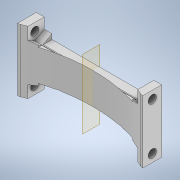
# Autodesk Inventor part: InnerSpacer
Saved by Autodesk Inventor 2020 (Build 240168000, 168)
## iProperties
Created: 2020-02-08
Part Number: InnerSpacer
Material: Generic
Document SubType Name: Modeling
Designer: srini
Density: 1 g/cm^3
Appearance: Default
Author: srini
Autodesk Inventor part; units mm, degrees
ref_plane "YZ Plane" through (0, 0, 0) normal (1, 0, 0) x (0, 1, 0)
ref_plane "XZ Plane" through (0, 0, 0) normal (0, 1, 0) x (-1, 0, 0)
ref_plane "XY Plane" through (0, 0, 0) normal (0, 0, 1) x (1, 0, 0)
sketch "Sketch1" plane through (0, 0, 0) normal (0, 0, 1) x (1, 0, 0)
  line L0 (-50.8, 12.7) -> (50.8, 12.7)
  line L1 (50.8, 12.7) -> (50.8, -12.7)
  line L2 (50.8, -12.7) -> (-50.8, -12.7)
  line L3 (-50.8, -12.7) -> (-50.8, 12.7)
  line L4 (-50.8, 25.4) -> (-38.1, 25.4)
  line L5 (-38.1, 25.4) -> (-38.1, 12.7)
  line L6 (-38.1, 12.7) -> (-50.8, 12.7)
  line L7 (-50.8, 12.7) -> (-50.8, 25.4)
  line L8 (-50.8, -12.7) -> (-38.1, -12.7)
  line L9 (-38.1, -12.7) -> (-38.1, -25.4)
  line L10 (-38.1, -25.4) -> (-50.8, -25.4)
  line L11 (-50.8, -25.4) -> (-50.8, -12.7)
  line L12 (38.1, 25.4) -> (50.8, 25.4)
  line L13 (50.8, 25.4) -> (50.8, 12.7)
  line L14 (50.8, 12.7) -> (38.1, 12.7)
  line L15 (38.1, 12.7) -> (38.1, 25.4)
  line L16 (38.1, -12.7) -> (50.8, -12.7)
  line L17 (50.8, -12.7) -> (50.8, -25.4)
  line L18 (50.8, -25.4) -> (38.1, -25.4)
  line L19 (38.1, -25.4) -> (38.1, -12.7)
  point P0 (0, 0)
  point P1 (-38.1, -12.7)
  point P2 (38.1, -12.7)
  dimension "d0" = 101.6
  dimension "d1" = 50.8
  dimension "d2" = 25.4
  dimension "d3" = 12.7
  dimension "d4" = 12.7
  dimension "d5" = 12.7
  constraints: 40 end point, 10 parallel, 7 collinear, 6 equal length, 5 horizontal, 5 perpendicular, 1 point on line
  measures "d0" distance of L0.start L0.end
  measures "d1" distance from line of point (0, 0) L3
  measures "d2" distance between parallel lines of L2 L0
  measures "d3" distance from line of point (0, 0) L0
  measures "d4" distance of L4.start L4.end
  measures "d5" distance of L6.end L4.start
extrude "Extrusion1" add sketch "Sketch1" along normal blind 15.24
sketch "Sketch2" plane through (50.8, -25.4, 0) normal (1, 0, 0) x (0, 0, -1)
  circle A0 centre (-7.62, 44.45) radius 3.3734
  line L0 (0, 0) -> (0, 50.8) projected
  line L1 (0, 50.8) -> (-15.24, 50.8) projected
  circle A1 centre (-7.62, 6.35) radius 3.3734
  point P0 (0, 25.4)
  dimension "d8" = 7.62
  dimension "d9" = 6.35
  dimension "d10" = 6.7469
  dimension "d13" = 38.1
  constraints: 2 centre point, 1 vertical, 2 other
  measures "d8" distance from line of A0.centre L0
  measures "d9" distance from line of A0.centre L1
  measures "d10" diameter of A0
  measures "d13" distance of A0.centre A1.centre
extrude "Extrusion2" cut sketch "Sketch2" against normal through all
sketch "Sketch3" plane through (-38.1, 12.7, 0) normal (1, 0, 0) x (0, 0, -1)
  circle A0 centre (-7.62, 6.35) radius 3.3734 projected
  circle A1 centre (-7.62, -31.75) radius 3.3734 projected
  line L0 (-7.62, 12.9967) -> (-1.8638, 9.6734)
  line L1 (-1.8638, 9.6734) -> (-1.8638, 3.0266)
  line L2 (-1.8638, 3.0266) -> (-7.62, -0.2967)
  line L3 (-7.62, -0.2967) -> (-13.3762, 3.0266)
  line L4 (-13.3762, 3.0266) -> (-13.3763, 9.6734)
  line L5 (-13.3763, 9.6734) -> (-7.62, 12.9967)
  line L6 (-7.62, -25.1033) -> (-1.8638, -28.4266)
  line L7 (-1.8638, -28.4266) -> (-1.8638, -35.0734)
  line L8 (-1.8638, -35.0734) -> (-7.62, -38.3967)
  line L9 (-7.62, -38.3967) -> (-13.3762, -35.0734)
  line L10 (-13.3762, -35.0734) -> (-13.3762, -28.4266)
  line L11 (-13.3762, -28.4266) -> (-7.62, -25.1033)
  point P0 (0, -12.7)
  point P1 (-7.62, 6.35)
  point P2 (-7.62, -31.75)
  dimension "d20" = 11.5125
  constraints: 24 end point, 2 coincident, 1 equal length, 1 vertical, 1 vertical alignment, 26 other
  measures "d20" distance between parallel lines of L4 L1
extrude "Extrusion3" cut sketch "Sketch3" against normal blind 6.35 contours A0 | A1 | L0 L1 L2 L3 L4 L5 | L6 L7 L8 L9 L10 L11
ref_plane "Work Plane1" through (0, -25.4, 0) normal (1, 0, 0) x (0, 0, -1)
mirror "Mirror1" about plane through (0, -25.4, 0) normal (1, 0, 0) of "Extrusion3"
sketch "Sketch4" plane through (-38.1, -12.7, 0) normal (0, -1, 0) x (1, 0, 0)
  circle A0 centre (38.1, 132.08) radius 127
  line L0 (0, 0) -> (76.2, 0) projected
  point P0 (38.1, 0)
  point P1 (38.1, 0)
  dimension "d23" = 132.08
  dimension "d24" = 254
  constraints: 1 centre point, 1 midpoint, 1 vertical alignment
  measures "d23" distance of point (38.1, 0) A0.centre
  measures "d24" diameter of A0
extrude "Extrusion4" cut sketch "Sketch4" against normal through all both and the other way through all
fillet "Fillet1" radius 6.35 2 edges at (49.7736, 0, 15.24) (-49.7736, 0, 15.24)
sketch "Sketch5" plane through (0, 0, 0) normal (0, 0, -1) x (-1, 0, 0)
  line L0 (-25.4, 9.525) -> (25.4, 9.525) construction
  line L1 (25.4, 9.525) -> (25.4, -9.525) construction
  line L2 (25.4, -9.525) -> (-25.4, -9.525) construction
  line L3 (-25.4, -9.525) -> (-25.4, 9.525) construction
  spline S0 degree 2 poles (-27.0681, 4.7718) (-25.0031, 4.7718) (-22.4544, 2.2603) (-22.4544, -0.0279) knots 0 0 0 1 2 2 2
  line L4 (-22.4544, -0.0279) -> (-22.4544, -9.9064)
  line L5 (-22.4544, -9.9064) -> (-24.4822, -9.9064)
  line L6 (-24.4822, -9.9064) -> (-24.4822, -0.1953)
  spline S1 degree 2 poles (-24.4822, -0.1953) (-24.4822, 1.4976) (-26.0635, 3.1347) (-27.496, 3.1347) knots 0 0 0 1 2 2 2
  spline S2 degree 2 poles (-27.496, 3.1347) (-30.0261, 3.1347) (-31.6074, 0.5674) knots 0 0 0 1 1 1
  line L7 (-31.6074, 0.5674) -> (-31.6074, -9.9064)
  line L8 (-31.6074, -9.9064) -> (-33.6166, -9.9064)
  line L9 (-33.6166, -9.9064) -> (-33.6166, 10.2412)
  line L10 (-33.6166, 10.2412) -> (-31.6074, 10.2412)
  line L11 (-31.6074, 10.2412) -> (-31.6074, 2.6138)
  spline S3 degree 2 poles (-31.6074, 2.6138) (-29.9703, 4.7718) (-27.0681, 4.7718) knots 0 0 0 1 1 1
  line L12 (-7.7019, -4.0277) -> (-15.1247, -4.0277)
  line L13 (-15.1247, -4.0277) -> (-16.985, -9.9064)
  line L14 (-16.985, -9.9064) -> (-19.0686, -9.9064)
  line L15 (-19.0686, -9.9064) -> (-12.8364, 9.1436)
  line L16 (-12.8364, 9.1436) -> (-10.0273, 9.1436)
  line L17 (-10.0273, 9.1436) -> (-3.6091, -9.9064)
  line L18 (-3.6091, -9.9064) -> (-5.7299, -9.9064)
  line L19 (-5.7299, -9.9064) -> (-7.7019, -4.0277)
  line L20 (-14.6038, -2.3347) -> (-8.2414, -2.3347)
  line L21 (-8.2414, -2.3347) -> (-11.4598, 7.6553)
  line L22 (-11.4598, 7.6553) -> (-14.6038, -2.3347)
  line L23 (10.9761, 7.5995) -> (0.9488, -8.2135)
  line L24 (0.9488, -8.2135) -> (11.1993, -8.2135)
  line L25 (11.1993, -8.2135) -> (11.1993, -9.9064)
  line L26 (11.1993, -9.9064) -> (-1.3209, -9.9064)
  line L27 (-1.3209, -9.9064) -> (-1.3209, -8.3065)
  line L28 (-1.3209, -8.3065) -> (8.725, 7.4879)
  line L29 (8.725, 7.4879) -> (-0.893, 7.4879)
  line L30 (-0.893, 7.4879) -> (-0.893, 9.1436)
  line L31 (-0.893, 9.1436) -> (10.9761, 9.1436)
  line L32 (10.9761, 9.1436) -> (10.9761, 7.5995)
  line L33 (17.878, 7.4879) -> (17.878, 0.7348)
  line L34 (17.878, 0.7348) -> (25.5426, 0.7348)
  line L35 (25.5426, 0.7348) -> (25.5426, -0.9581)
  line L36 (25.5426, -0.9581) -> (17.878, -0.9581)
  line L37 (17.878, -0.9581) -> (17.878, -8.2507)
  line L38 (17.878, -8.2507) -> (26.1379, -8.2507)
  line L39 (26.1379, -8.2507) -> (26.1379, -9.9064)
  line L40 (26.1379, -9.9064) -> (15.8316, -9.9064)
  line L41 (15.8316, -9.9064) -> (15.8316, 9.1436)
  line L42 (15.8316, 9.1436) -> (26.1379, 9.1436)
  line L43 (26.1379, 9.1436) -> (26.1379, 7.4879)
  line L44 (26.1379, 7.4879) -> (17.878, 7.4879)
  spline S4 degree 2 poles (32.8538, -7.2647) (32.8538, -7.9716) (33.4119, -8.5669) (34.0072, -8.5669) knots 0 0 0 1 2 2 2
  spline S5 degree 2 poles (34.0072, -8.5669) (34.4351, -8.5669) (34.8444, -8.4553) knots 0 0 0 1 1 1
  line L45 (34.8444, -8.4553) -> (35.1234, -9.9064)
  spline S6 degree 2 poles (35.1234, -9.9064) (34.3235, -10.2412) (33.4863, -10.2412) knots 0 0 0 1 1 1
  spline S7 degree 2 poles (33.4863, -10.2412) (32.2585, -10.2412) (30.8446, -8.846) (30.8446, -7.5623) knots 0 0 0 1 2 2 2
  line L46 (30.8446, -7.5623) -> (30.8446, 10.2412)
  line L47 (30.8446, 10.2412) -> (32.8538, 10.2412)
  line L48 (32.8538, 10.2412) -> (32.8538, -7.2647)
  point P0 (0, 0)
  dimension "d2" = 25.4
  dimension "d30" = 50.8
  dimension "d31" = 25.4
  dimension "d32" = 19.05
  dimension "d33" = 9.525
  constraints: 2 other
  measures "d30" distance of L0.start L0.end
  measures "d31" distance from line of point (0, 0) L3
  measures "d32" distance of L0.end L1.end
  measures "d33" distance from line of point (0, 0) L0
emboss "Emboss1" sketch "Sketch5" operation cut depth 0.9 direction (0, 0, 1)
sketch "Sketch6" plane through (44.45, 15.7266, 13.3762) normal (-1, 0, 0) x (0, 1, 0)
  point P0 (-15.7266, 13.3762)
sketch "Sketch7" plane through (-44.45, 12.7, 0) normal (1, 0, 0) x (0, 0, -1)
  line L0 (-7.62, -0.2967) -> (-18.6172, 6.0525)
  line L1 (-18.6172, 6.0525) -> (-19.0863, 27.5679)
  line L2 (-19.0863, 27.5679) -> (7.0141, 38.5627)
  line L3 (7.0141, 38.5627) -> (10.8216, 10.3505)
  line L4 (10.8216, 10.3505) -> (-7.62, -0.2967)
  line L5 (-7.62, -0.2967) -> (-13.3762, 3.0266) projected
  line L6 (-1.8638, 3.0266) -> (-7.62, -0.2967) projected
  line L7 (-7.62, -25.1033) -> (3.6671, -31.6199)
  line L8 (3.6671, -31.6199) -> (4.0138, -47.5222)
  line L9 (4.0138, -47.5222) -> (-21.2734, -46.4313)
  line L10 (-21.2734, -46.4313) -> (-22.1804, -33.5097)
  line L11 (-22.1804, -33.5097) -> (-7.62, -25.1033)
  line L12 (-7.62, -25.1033) -> (-1.8638, -28.4266) projected
  line L13 (-13.3762, -28.4266) -> (-7.62, -25.1033) projected
  point P0 (0, -12.7)
  constraints: 20 end point, 4 collinear
extrude "Extrusion5" cut sketch "Sketch7" along normal up to surface (88.9 mm away)
equation "\"d1\" = 0.5 * d0"
equation "\"d3\" = 0.5 * d2"
equation "\"d8\" = 0.5 * d6"
equation "\"d31\" = 0.5 * d30"
equation "\"d33\" = 0.5 * d32"
equation "\"d6\" = 15.24"
body "Solid1"
